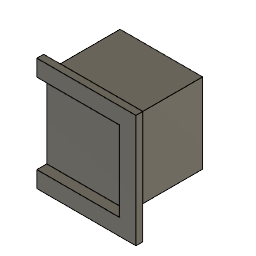
Spacer for Display (Autodesk Fusion 360 design; units mm, degrees)
Autodesk Fusion 360 part; units mm, degrees
sketch "Sketch1" plane through (0, 0, 0) normal (0, 1, 0) x (1, 0, 0)
  line L0 (0, 0) -> (12.5, 0)
  line L1 (12.5, 0) -> (12.5, -12.1)
  line L2 (12.5, -12.1) -> (0, -12.1)
  line L3 (0, -12.1) -> (0, 0)
  line L4 (0, -12.1) -> (0, -14.6)
  line L5 (0, -14.6) -> (15, -14.6)
  line L6 (15, -14.6) -> (15, 0.0553)
  line L7 (15, 0.0553) -> (15, 2.5)
  line L8 (15, 2.5) -> (0, 2.5)
  line L9 (0, 2.5) -> (0, 0)
  dimension "d1" = 12.1
  dimension "d2" = 12.5
  dimension "d3" = 2.5
  dimension "d4" = 2.5
  dimension "d5" = 2.5
  constraint horizontal L0
  constraint vertical L1
  constraint horizontal L2
  constraint vertical L3
  constraint coincident L0.start L3.end
  constraint perpendicular L2 L4
  constraint perpendicular L4 L5
  constraint perpendicular L5 L6
  constraint perpendicular L0 L7
  constraint perpendicular L7 L8
  constraint parallel L6 L9
  measures "d1" distance of L0.end L1.end
  measures "d2" distance of L1.end L2.end
  measures "d3" distance of L2 L5
  measures "d4" distance of L0 L8
  measures "d5" distance of L1 L6
extrude "Extrude1" add sketch "Sketch1" along normal blind 11.1 contours L0 L1 L2 L3
extrude "Extrude3" add sketch "Sketch1" along normal blind -1.5 and the other way blind -2 contours L0 L1 L2 L4 L5 L6 L7 L8 L9
chamfer "Chamfer2" distance 2.461 angle 45 3 edges at (7.5, 2, 14.6) (15, 2, 6.05) (7.5, 2, -2.5)
